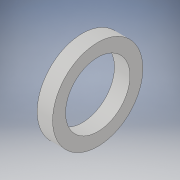
# Autodesk Inventor part: BT306_trajan20_21
Saved by Autodesk Inventor 2022.2 (Build 262287000, 287)
## iProperties
Company: HTBLA Kaindorf
RuleStatus: InUse
Created: 2022-09-14
Part Number: BT306_trajan20_21
Project: Zeichenmaschine_v2_a
Material: Generisch
Description: beilagscheibe
Document SubType Name: Modeling
Designer: trajan20
Density: 1 g/cm^3
Appearance: Vorgabe
Mass: 0.0226195 g
Surface Area: 0.82938 cm^2
Volume: 0.0226195 cm^3
AfterDocNew0: iProperties-Editor_aufrufen
Author: jan
Keywords: 2021
Autodesk Inventor part; units mm, degrees
ref_plane "YZ Plane" through (0, 0, 0) normal (1, 0, 0) x (0, 1, 0)
ref_plane "XZ Plane" through (0, 0, 0) normal (0, 1, 0) x (-1, 0, 0)
ref_plane "XY Plane" through (0, 0, 0) normal (0, 0, 1) x (1, 0, 0)
sketch "Skizze3" plane through (0, 0, 0) normal (0, 0, 1) x (1, 0, 0)
  line L0 (2.5, 0) -> (2.5, 1.2)
  line L1 (2.5, 1.2) -> (3.5, 1.2)
  line L2 (3.5, 1.2) -> (3.5, 0)
  line L3 (3.5, 0) -> (2.5, 0)
  line L4 (0, -2.096) -> (0, 2.197)
  point P0 (0, 0)
  dimension "d5" = 5
  dimension "d6" = 7
  dimension "d7" = 1.2
  constraints: 10 end point, 3 perpendicular, 2 point on line, 2 vertical
  measures "d5" diameter of L0 L4
  measures "d6" diameter of L2 L4
  measures "d7" distance between parallel lines of L3 L1
revolve "Umdrehung1" add sketch "Skizze3" angle 360 about axis through (0, -2.096, 0) along (0, -1, 0)
